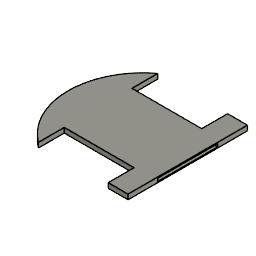
BottomFront (Autodesk Fusion 360 design; units mm, degrees)
part number: 2026-01-06-12-46-14-723
Autodesk Fusion 360 part; units mm, degrees
sketch "Bottom front base" plane through (0, 0, 0) normal (0, 0, 1) x (1, 0, 0)
  line L0 (40, 60) -> (60, 60)
  line L1 (60, 60) -> (60, -60)
  line L2 (60, -60) -> (40, -60)
  line L3 (60, 0) -> (57.5, 0) construction
  line L4 (57.5, -60) -> (57.5, -6) construction
  line L5 (57.5, -6) -> (-12.5, -6) construction
  line L6 (-12.5, -6) -> (-12.5, -34) construction
  line L7 (-12.5, -34) -> (-30, -34)
  line L8 (-12.5, -34) -> (40, -34)
  line L9 (40, -34) -> (40, -60)
  line L10 (-30, -34) -> (-30, -60)
  arc A0 (-30, 60) -> (-30, -60) centre (15, 0) ccw
  line L11 (-30, 34) -> (-30, 60)
  line L12 (-12.5, 34) -> (40, 34)
  line L13 (-12.5, 34) -> (-30, 34)
  line L14 (40, 34) -> (40, 60)
  dimension "d1" = 120
  dimension "d3" = 2.5
  dimension "d4" = 54
  dimension "d5" = 70
  dimension "d6" = 28
  dimension "d9" = 70
  constraint horizontal L0
  constraint perpendicular L0 L1
  constraint parallel L0 L2
  constraint midpoint L1 L3.start
  constraint perpendicular L1 L3
  constraint coincident L2 L4.start
  constraint perpendicular L2 L4
  constraint perpendicular L4 L5
  constraint perpendicular L5 L6
  constraint perpendicular L6 L7
  constraint perpendicular L6 L8
  constraint perpendicular L2 L9
  constraint perpendicular L2 L10
  constraint symmetric L3 L6.end L12.start
  constraint symmetric L3 L7.end L11.start
  constraint symmetric L3 L8.end L12.end
  constraint symmetric L3 L2.end L0.start
  constraint symmetric L3 L10.end A0.start
  measures "d1" distance of L0.end L1.end
  measures "d3" distance of L3.start L3.end
  measures "d4" distance of L4.start L4.end
  measures "d5" distance of L4.end L5.end
  measures "d6" distance of L5.end L6.end
  measures "d9" distance of L7.end L8.end
extrude "Bottom front height" add sketch "Bottom front base" along normal blind 5
sketch "Connector hole" plane through (60, 0, 0) normal (1, 0, 0) x (0, 1, 0)
  line L0 (-60, 0) -> (60, 0)
  line L1 (60, 0) -> (60, 5)
  line L2 (60, 5) -> (-60, 5)
  line L3 (-60, 5) -> (-60, 0)
  line L4 (0, 0) -> (0, -0.1551)
  line L5 (0, 0) -> (0, 5) construction
  line L6 (30, 4) -> (-30, 4)
  line L7 (-30, 4) -> (-30, 1)
  line L8 (-30, 1) -> (30, 1)
  line L9 (30, 1) -> (30, 4)
  line L10 (30, 4) -> (-30, 1) construction
  line L11 (-30, 4) -> (30, 1) construction
  point P0 (0, 2.5)
  dimension "d12" = 3
  dimension "d13" = 60
  constraint coincident L4.start L5.start
  constraint perpendicular L0 L4
  constraint midpoint L2 L5.end
  constraint horizontal L6
  constraint perpendicular L6 L7
  constraint parallel L6 L8
  constraint parallel L7 L9
  constraint coincident L10 P0
  constraint coincident L11 P0
  constraint midpoint L5 P0
  measures "d12" distance of L6.end L7.end
  measures "d13" distance of L6.start L6.end
extrude "Connector hole (1)" cut sketch "Connector hole" against normal blind 60 contours L6 L7 L8 L9
equation "d6 = 54 mm - 26 mm"
named bodies: "Bottom front"
